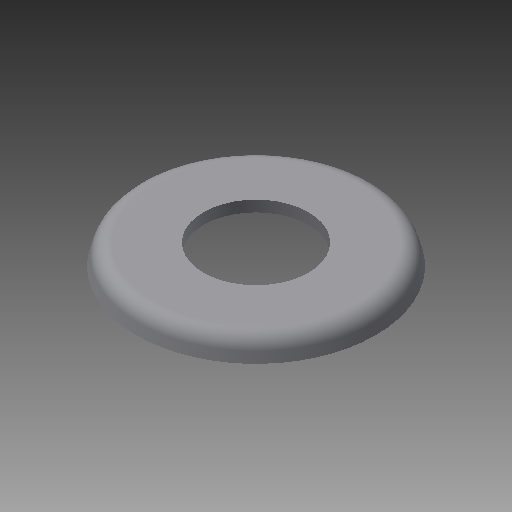
# Autodesk Inventor part: Rondella superiore
Saved by Autodesk Inventor 2019 (Build 230136000, 136)
## iProperties
Created: 2011-09-21
Part Number: Rondella superiore
Document SubType Name: Modeling
Designer: Stefano
Density: 1 g/cm^3
Material: 一般
Appearance: 既定
Author: Stefano
Autodesk Inventor part; units mm, degrees
ref_plane "YZ Plane" through (0, 0, 0) normal (1, 0, 0) x (0, 1, 0)
ref_plane "XZ Plane" through (0, 0, 0) normal (0, 1, 0) x (-1, 0, 0)
ref_plane "XY Plane" through (0, 0, 0) normal (0, 0, 1) x (1, 0, 0)
sketch "Schizzo1" plane through (0, 0, 0) normal (0, 0, 1) x (1, 0, 0)
  line L0 (4.75, 6.5534) -> (9.25, 6.5534)
  arc A0 (10.6023, 5.5157) -> (9.25, 6.5534) centre (9.25, 5.1534) ccw
  line L1 (4.75, 5.5534) -> (9.25, 5.5534)
  line L2 (4.75, 5.5534) -> (4.75, 6.5534)
  line L3 (0, 6.5534) -> (0, 3.993) construction
  arc A1 (9.6364, 5.2569) -> (9.25, 5.5534) centre (9.25, 5.1534) ccw
  line L4 (9.8599, 4.4226) -> (10.8258, 4.6814)
  line L5 (10.6023, 5.5157) -> (10.8258, 4.6814)
  line L6 (9.8599, 4.4226) -> (9.6364, 5.2569)
  point P0 (0, 0)
  dimension "d1" = 4.5
  dimension "d2" = 1
  dimension "d8" = 4.75
  dimension "d10" = 0.4
  dimension "d11" = 9.25
  constraints: 14 end point, 4 point on circle, 4 tangent, 3 parallel, 2 centre point, 2 perpendicular, 1 vertical alignment
  measures "d1" distance of L0.start L0.end
  measures "d2" distance between parallel lines of L0 L1
  measures "d8" distance between parallel lines of L2 L3
  measures "d10" radius of A1
  measures "d11" distance from line of L1.end L3
revolve "Rivoluzione1" add sketch "Schizzo1" angle 360 about axis through (0, 6.5534, 0) along (0, -1, 0)
